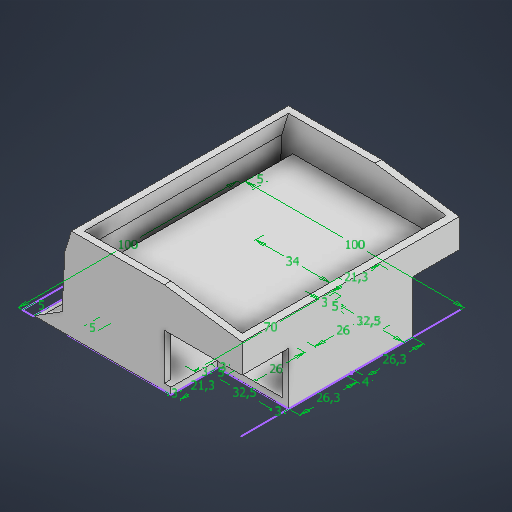
# Autodesk Inventor part: Peça1
Saved by Autodesk Inventor 2026 (Build 300175050, 175E)
## iProperties
Created: 2025-11-08
Part Number: Peça1
Material: Genérico
Document SubType Name: Modeling
Designer: luzjl
Density: 1 g/cm^3
Appearance: Padrão
Author: luzjl
Autodesk Inventor part; units mm, degrees
ref_plane "YZ Plane" through (0, 0, 0) normal (1, 0, 0) x (0, 1, 0)
ref_plane "XZ Plane" through (0, 0, 0) normal (0, 1, 0) x (-1, 0, 0)
ref_plane "XY Plane" through (0, 0, 0) normal (0, 0, 1) x (1, 0, 0)
sketch "Esboço1" plane through (0, 0, 0) normal (0, 1, 0) x (-1, 0, 0)
  line L0 (50, 50) -> (50, -50)
  line L1 (-50, -50) -> (-50, 50)
  line L2 (-50, -2) -> (-50, 2)
  line L3 (-50, -2) -> (-50, -28.3)
  line L4 (-50, 2) -> (-50, 28.3)
  line L5 (-50, 28.3) -> (-17.5, 28.3)
  line L6 (-50, -28.3) -> (-17.5, -28.3)
  line L7 (-17.5, -28.3) -> (-17.5, -49.6)
  line L8 (-17.5, 28.3) -> (-17.5, 49.6)
  line L9 (-39.9, -28.3) -> (-27.6, -28.3)
  line L10 (-27.6, -28.3) -> (-27.6, -2.3)
  line L11 (-27.6, -2.3) -> (-39.9, -2.3)
  line L12 (-39.9, -2.3) -> (-39.9, -28.3)
  line L13 (-27.6, 28.3) -> (-27.6, 2.3)
  line L14 (-27.6, 2.3) -> (-39.9, 2.3)
  line L15 (-39.9, 2.3) -> (-39.9, 28.3)
  line L16 (50, 50) -> (45, 50)
  line L17 (50, -50) -> (45, -50)
  line L18 (45, 50) -> (45, -50)
  line L19 (-17.5, -28.3) -> (-14.5, -28.3)
  line L20 (-14.5, -49.6) -> (-17.5, -49.6)
  line L21 (-17.5, 28.3) -> (-14.5, 28.3)
  line L22 (-14.5, 49.6) -> (-17.5, 49.6)
  line L23 (-9.5, -35) -> (-9.5, 35)
  line L24 (-9.5, -35) -> (24.5, -35)
  line L25 (24.5, -35) -> (24.5, 35)
  line L26 (24.5, 35) -> (-9.5, 35)
  line L27 (29.5, 35) -> (29.5, -35)
  line L28 (-14.5, 49.6) -> (29.5, 49.6)
  line L29 (29.5, 49.6) -> (29.5, -49.6)
  line L30 (29.5, -49.6) -> (-14.5, -49.6)
  line L31 (26.5, -46.6) -> (26.5, 46.6)
  line L32 (-14.5, -28.3) -> (-17.5, -28.3)
  line L33 (-14.5, -28.3) -> (-14.5, -46.6)
  line L34 (-14.5, 46.6) -> (-14.5, 28.3)
  line L35 (26.5, -46.6) -> (-14.5, -46.6)
  line L36 (26.5, 46.6) -> (-14.5, 46.6)
  line L37 (-50, 28.3) -> (-47, 28.3)
  line L38 (-47, 28.3) -> (-47, -28.3)
  line L39 (-14.5, -28.3) -> (-14.5, -25.3)
  line L40 (-14.5, -25.3) -> (-17.5, -25.3)
  line L41 (-17.5, -25.3) -> (-22.5, -25.3)
  line L42 (-22.5, -25.3) -> (-22.5, -28.3)
  line L43 (-14.5, 28.3) -> (-14.5, 25.3)
  line L44 (-14.5, 25.3) -> (-17.5, 25.3)
  line L45 (-17.5, 25.3) -> (-22.5, 25.3)
  line L46 (-22.5, 25.3) -> (-22.5, 28.3)
  point P0 (0, 0)
  point P1 (-50, 0)
  point P2 (-33.75, -28.3)
  dimension "d0" = 100
  dimension "d1" = 100
  dimension "d2" = 4
  dimension "d3" = 26.3
  dimension "d4" = 26.3
  dimension "d5" = 32.5
  dimension "d6" = 32.5
  dimension "d7" = 21.3
  dimension "d8" = 21.3
  dimension "d9" = 12.3
  dimension "d10" = 26
  dimension "d11" = 26
  dimension "d12" = 5
  dimension "d13" = 5
  dimension "d14" = 3
  dimension "d15" = 3
  dimension "d17" = 70
  dimension "d18" = 34
  dimension "d19" = 5
  dimension "d20" = 3
  dimension "d23" = 3
  dimension "d42" = 5
  dimension "d43" = 3
  dimension "d44" = 5
  constraints: 94 end point, 21 point on line, 11 perpendicular, 6 vertical, 5 horizontal, 4 midpoint, 3 parallel
  measures "d0" distance of L0.end L1.start
  measures "d1" distance of L0.start L0.end
  measures "d2" distance of L2.start L2.end
  measures "d3" distance of L2.start L3.end
  measures "d4" distance of L2.end L4.end
  measures "d5" distance of L4.end L5.end
  measures "d6" distance of L3.end L6.end
  measures "d7" distance of L6.end L7.end
  measures "d8" distance of L5.end L8.end
  measures "d9" distance of L9.start L9.end
  measures "d10" distance of L9.end L10.end
  measures "d11" distance of L13.start L13.end
  measures "d12" distance of L0.start L16.end
  measures "d13" distance of L0.end L17.end
  measures "d14" distance of L6.end L19.end
  measures "d15" distance of L5.end L21.end
  measures "d17" distance of L23.start L23.end
  measures "d18" distance of L23.start L24.end
  measures "d19" distance of L25.end L27.start
  measures "d20" distance of L22.start L34.start
  measures "d23" distance of L4.end L37.end
  measures "d42" distance of L40.end L41.end
  measures "d43" distance of L21.end L43.end
  measures "d44" distance of L44.end L45.end
extrude "Extrusão1" add sketch "Esboço1" along normal blind 3 contours L38 L5 L15 L14 L13 L46 L45 L44 L43 L34 L36 L31 L35 L33 L39 L40 L41 L42 L6 L10 L11 L12 | L12 L11 L10 L6 | L5 L13 L14 L15 | L42 L41 L40 L39 L19 L6 | L5 L21 L43 L44 L45 L46 | L23 L26 L25 L24
extrude "Extrusão2" add sketch "Esboço1" along normal blind 27 contours L1 L5 L38 L6
sketch "Esboço2" plane through (14.5, 0, -46.6) normal (0, 0, -1) x (-1, 0, 0)
  line L0 (41, 0) -> (0, 0) projected
  line L1 (41, 0) -> (59.5, 0)
  line L2 (41, 0) -> (41, 3) projected
  line L3 (41, 0) -> (41, 3)
  line L4 (41, 3) -> (0, 3) projected
  line L5 (-32.5, 3) -> (0, 3) projected
  line L6 (-32.5, 3) -> (-32.5, 27) projected
  line L7 (-32.5, 27) -> (-32.5, 24)
  line L8 (-32.5, 27) -> (3, 27)
  line L9 (3, 27) -> (3, 24)
  line L10 (3, 24) -> (-32.5, 24)
  line L11 (0, 3) -> (0, 27)
  line L12 (0, 3) -> (3, 3)
  line L13 (3, 3) -> (37, 3)
  line L14 (0, 3) -> (-35.5, 3)
  line L15 (-35.5, 0) -> (-35.5, 27) projected
  line L16 (-11.75, 3) -> (-23.75, 3)
  line L17 (-23.75, 3) -> (-23.75, 15)
  line L18 (-23.75, 15) -> (-11.75, 15)
  line L19 (-11.75, 15) -> (-11.75, 3)
  line L20 (3, 3) -> (3, 21)
  line L21 (0, 27) -> (0, 42)
  line L22 (37, 3) -> (37, 21)
  line L23 (37, 21) -> (3, 21)
  line L24 (41, 3) -> (55.9231, 3)
  line L25 (0, 3) -> (41, 3) projected
  line L26 (-32.5, 27) -> (-35.5, 27) projected
  line L27 (-32.5, 27) -> (37.5, 27)
  line L28 (0, 42) -> (38, 42)
  line L29 (0, 42) -> (39.5, 42)
  line L30 (39.5, 42) -> (42.5, 32.2)
  line L31 (3, 24) -> (37.5, 24)
  line L32 (37.5, 24) -> (37.5, 27)
  line L33 (-23.75, 3) -> (-11.75, 15)
  line L34 (-23.75, 15) -> (-11.75, 3)
  line L35 (42.5, 3) -> (44, 3)
  line L36 (44, 3) -> (42.5, 32.2)
  line L37 (59.5, 0) -> (57, 0)
  line L38 (-17.75, 24) -> (-17.75, 3)
  line L39 (0, 27) -> (0, 37)
  line L40 (-35.5, 27) -> (-35.5, 32)
  line L41 (39.5, 42) -> (42.5, 42)
  line L42 (42.5, 32.2) -> (45.5, 32.2)
  line L43 (43.7518, 7.8322) -> (46.7478, 7.9861)
  line L44 (45.5, 32.2) -> (42.5, 42)
  line L45 (45.5, 32.2) -> (46.7478, 7.9861)
  line L46 (59.5, 0) -> (62, 0)
  line L47 (59.5, 0) -> (46.7478, 7.9861)
  line L48 (0, 42) -> (-35.5, 37.1)
  line L49 (-35.5, 37.1) -> (-35.5, 32)
  point P0 (14.5, 0)
  point P1 (0, 24)
  point P2 (54.7096, 3)
  dimension "d28" = 18.5
  dimension "d31" = 3
  dimension "d32" = 35.5
  dimension "d33" = 3
  dimension "d34" = 34
  dimension "d35" = 12
  dimension "d36" = 12
  dimension "d37" = 18
  dimension "d38" = 15
  dimension "d50" = 18
  dimension "d55" = 70
  dimension "d57" = 38
  dimension "d61" = 1.5
  dimension "d62" = 2.5
  dimension "d63" = 10
  dimension "d64" = 5
  dimension "d65" = 3
  dimension "d66" = 3
  dimension "d67" = 3
  dimension "d68" = 2.5
  constraints: 84 end point, 16 point on line, 11 perpendicular, 6 horizontal, 2 collinear, 2 midpoint, 2 vertical
  measures "d28" distance of L0.start L1.end
  measures "d31" distance of L6.end L7.end
  measures "d32" distance of L6.end L8.end
  measures "d33" distance of L4.end L12.end
  measures "d34" distance of L12.end L13.end
  measures "d35" distance of L16.start L16.end
  measures "d36" distance of L16.end L17.end
  measures "d37" distance of L12.end L20.end
  measures "d38" distance of L11.end L21.end
  measures "d50" distance of L13.end L22.end
  measures "d55" distance of L6.end L27.end
  measures "d57" distance of L21.end L28.end
  measures "d61" distance of L35.start L35.end
  measures "d62" distance of L1.end L37.end
  measures "d63" distance of L11.end L39.end
  measures "d64" distance of L15.end L40.end
  measures "d65" distance of L29.end L41.end
  measures "d66" distance of L30.end L42.end
  measures "d67" distance of L43.start L43.end
  measures "d68" distance of L1.end L46.end
extrude "Extrusão3" add sketch "Esboço1" along normal blind 3 contours L19 L33 L35 L31 L36 L34 L21 L8 L22 L28 L29 L27 L30 L20 L7
extrude "Extrusão7" add sketch "Esboço2" along normal blind 3 contours L2 L24 L47 L1 | L4 L22 L23 L20 L11 L10 L31 L32 L27 L8 L21 L28 L29 L30 L36 L24 | L4 L20 L23 L22 | L11 L8 L9 L10 | L10 L6 L8 L11 | L9 L27 L32 L31 | L8 L26 L40 L49 L48 L21
mirror "Espelhar2" about plane through (0, 0, 0) normal (0, 0, 1) of "Extrusão7"
sketch "Esboço4" plane through (14.5, 0, -46.6) normal (0, 0, 1) x (1, 0, 0)
  line L0 (32.5, 27) -> (-37.5, 27)
  line L1 (-37.5, 27) -> (-37.5, 24)
  line L2 (-37.5, 24) -> (32.5, 24)
  line L3 (32.5, 24) -> (32.5, 27)
  line L4 (32.5, 27) -> (35.5, 27)
  line L5 (35.5, 27) -> (35.5, 24)
  line L6 (35.5, 24) -> (32.5, 24)
  point P0 (-14.5, 0)
  dimension "d71" = 70
  dimension "d72" = 3
  dimension "d73" = 3
  dimension "d74" = 3
  constraints: 14 end point, 3 perpendicular, 2 point on line, 1 horizontal
  measures "d71" distance of L0.start L0.end
  measures "d72" distance of L0.end L1.end
  measures "d73" distance of L0.start L4.end
  measures "d74" distance of L4.end L5.end
extrude "Extrusão8" add sketch "Esboço4" along normal blind 96.2
sketch "Esboço5" plane through (14.5, 42, 46.6) normal (0, 0, -1) x (-1, 0, 0)
  line L0 (-32.5, -15) -> (-32.5, -18) projected
  line L1 (-32.5, -18) -> (-32.5117, -4.4875)
  line L2 (0, 0) -> (-35.5, -4.9) projected
  line L3 (-32.5117, -4.4875) -> (-35.5, -4.9)
  line L4 (-35.5, -18) -> (0, -18) projected
  line L5 (-35.5, -4.9) -> (-35.5, -18)
  line L6 (-35.5, -18) -> (-32.5, -18)
  point P0 (14.5, -42)
  constraints: 8 end point, 2 perpendicular, 1 collinear, 1 point on line
extrude "Extrusão9" add sketch "Esboço5" along normal blind 96.2
sketch "Esboço6" plane through (17.5, 0, -49.6) normal (0, 0, -1) x (-1, 0, 0)
  line L0 (42.5, 42) -> (3, 42) projected
  line L1 (42.5, 42) -> (45.5, 42)
  line L2 (47, 3) -> (45.5, 32.2) projected
  line L3 (45.5, 32.2) -> (48.5, 32.2)
  line L4 (46.7519, 7.8299) -> (49.7479, 7.9838)
  line L5 (57.7096, 3) -> (47, 3) projected
  line L6 (49.7479, 7.9838) -> (57.7096, 3)
  line L7 (49.7479, 7.9838) -> (48.5, 32.2)
  line L8 (45.5, 42) -> (48.5, 32.2)
  line L9 (45.5, 32.2) -> (42.5, 42) projected
  line L10 (42.5, 42) -> (45.5, 32.2)
  point P0 (17.5, 0)
  dimension "d79" = 3
  dimension "d80" = 3
  dimension "d81" = 3
  constraints: 14 end point, 2 horizontal, 1 collinear, 1 perpendicular, 1 point on line
  measures "d79" distance of L0.start L1.end
  measures "d80" distance of L2.end L3.end
  measures "d81" distance of L4.start L4.end
sketch "Esboço7" plane through (14.5, 0, -46.6) normal (0, 0, 1) x (1, 0, 0)
  line L0 (-44, 3) -> (-44, 0) projected
  line L1 (-44, 3) -> (-44, 0)
  line L2 (-54.7096, 3) -> (-44, 3) projected
  line L3 (-44, 3) -> (-54.7096, 3)
  line L4 (-59.5, 0) -> (-54.7096, 3) projected
  line L5 (-54.7096, 3) -> (-59.5, 0)
  line L6 (-59.5, 0) -> (-44, 0)
  point P0 (-14.5, 0)
  constraints: 8 end point, 2 collinear, 1 parallel, 1 vertical
extrude "Extrusão10" add sketch "Esboço7" along normal blind 96.2
extrude "Extrusão11" add sketch "Esboço6" against normal blind 99.2
